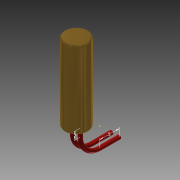
# Autodesk Inventor part: heater-cartrig
Saved by Autodesk Inventor 2015 (Build 190159000, 159)
## iProperties
Created: 2015-02-05
Part Number: heater-cartrig
Material: Типовые
Document SubType Name: Modeling
Designer: Parabolik
Density: 1 g/cm^3
Appearance: Латунь - сатинированная
Author: Parabolik
Autodesk Inventor part; units mm, degrees
ref_plane "XZ Plane" through (0, 0, 0) normal (0, 1, 0) x (-1, 0, 0)
sketch "Эскиз1" plane through (0, 0, 0) normal (0, 0, 1) x (1, 0, 0)
  circle A0 centre (0, 0) radius 3
  dimension "d0" = 6
  constraints: 1 centre point, 1 coincident
  measures "d0" diameter of A0
extrude "Выдавливание1" add sketch "Эскиз1" along normal blind 20
fillet "Сопряжение1" radius 0.5 2 edges at (-3, 0, 20) (-3, 0, 0)
sketch "Эскиз2" plane through (0, 0, 0) normal (0, 0, -1) x (-1, 0, 0)
  circle A0 centre (0, 0) radius 2.25
  circle A1 centre (1, 0) radius 0.5
  circle A2 centre (-1, 0) radius 0.5
  line L0 (0, 2.25) -> (0, -2.5)
  circle A3 centre (0, 0) radius 2.5 projected
  dimension "d4" = 4.5
  dimension "d5" = 1
  dimension "d6" = 1
  dimension "d7" = 2
  constraints: 2 centre point, 2 end point, 2 vertical alignment, 1 coincident, 1 symmetric about line, 1 vertical, 3 other
  measures "d5" diameter of A1
  measures "d6" diameter of A2
  measures "d7" distance of A1.centre A2.centre
extrude "Выдавливание2" cut sketch "Эскиз2" against normal blind 1 contours A0 L0 | L0 A0
ref_plane "РабПлоскость1" through (1, 0, 0) normal (1, 0, 0) x (0, 1, 0)
sketch "Эскиз3" plane through (1, 0, 0) normal (1, 0, 0) x (0, 1, 0)
  line L0 (0, 0) -> (0, -2)
  arc A0 (0, -2) -> (5.0002, -6.9531) centre (4.9534, -2) ccw
  line L1 (5.0002, -6.9531) -> (10.0002, -6.9531)
  dimension "d11" = 2
  dimension "d12" = 5
  constraints: 4 end point, 2 point on circle, 1 centre point, 1 horizontal, 1 tangent, 1 vertical
  measures "d11" distance of L0.start L0.end
  measures "d12" distance of L1.start L1.end
sketch "Эскиз4" plane through (1, 0, 0) normal (0, 0, -1) x (-1, 0, 0)
  circle A0 centre (0, 0) radius 0.5
  circle A1 centre (2, 0) radius 0.5 projected
  circle A2 centre (2, 0) radius 0.5
  point P0 (1, 0)
  constraints: 2 centre point, 1 coincident
sweep "Сдвиг1" add profiles "Эскиз4" path "Эскиз3" contours A0
ref_plane "РабПлоскость2" through (-1, 0, 0) normal (1, 0, 0) x (0, 1, 0)
sketch "Эскиз5" plane through (-1, 0, 0) normal (1, 0, 0) x (0, 1, 0)
  line L0 (0, 0) -> (0, -2)
  line L1 (-0.5, -2) -> (0.5, -2) projected
  line L2 (5.005, -7.4531) -> (4.9955, -6.4532) projected
  arc A0 (0, -2) -> (5.0002, -6.9531) centre (4.9076, -2.0462) ccw
  line L3 (5.0002, -6.9531) -> (10.0002, -6.9531)
  line L4 (10.0002, -7.4531) -> (10.0002, -6.4531) projected
  constraints: 4 end point, 3 midpoint, 2 point on circle, 1 centre point
sweep "Сдвиг2" add profiles "Эскиз4" path "Эскиз5" path curves L0 A0 L3 contours A1
